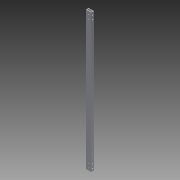
# Autodesk Inventor part: M - 26 inch rail
Saved by Autodesk Inventor 2013 (Build 170138000, 138)
## iProperties
Created: 2013-02-16
Part Number: M - 26 inch rail
Material: Aluminum 6061
Document SubType Name: Modeling
Designer: Moses
Mass: 356.175 g
Surface Area: 842.395 cm^2
Volume: 131.43 cm^3
Density: 2.71 g/cm^3
Author: Moses
Autodesk Inventor part; units mm, degrees
ref_plane "YZ Plane" through (0, 0, 0) normal (1, 0, 0) x (0, 1, 0)
ref_plane "XZ Plane" through (0, 0, 0) normal (0, 1, 0) x (-1, 0, 0)
sketch "Sketch1" plane through (0, 0, 0) normal (0, 1, 0) x (-1, 0, 0)
  line L0 (0, 0) -> (25.4, 0)
  line L1 (25.4, 0) -> (25.4, 12.7)
  line L2 (25.4, 12.7) -> (0, 12.7)
  line L3 (0, 12.7) -> (0, 0)
  line L4 (3.175, 9.525) -> (22.225, 9.525)
  line L5 (22.225, 9.525) -> (22.225, 3.175)
  line L6 (22.225, 3.175) -> (3.175, 3.175)
  line L7 (3.175, 3.175) -> (3.175, 9.525)
  dimension "d0" = 25.4
  dimension "d2" = 3.175
  dimension "d5" = 12.7
  constraints: 16 end point, 4 parallel, 2 perpendicular, 1 horizontal, 3 other
  measures "d0" distance of L1.end L2.end
  measures "d2" distance between parallel lines of L2 L4
  measures "d5" distance of L0.end L1.end
extrude "Extrusion1" add sketch "Sketch1" along normal blind 660.4
sketch "Sketch2" plane through (-25.4, 0, 12.7) normal (0, 0, 1) x (1, 0, 0)
  circle A0 centre (12.7, 41.275) radius 3.3782 projected
  circle A1 centre (12.7, 22.225) radius 3.3782 projected
  circle A2 centre (12.7, 619.125) radius 3.3782 projected
  circle A3 centre (12.7, 638.175) radius 3.3782 projected
  line L0 (25.4, 0) -> (0, 0) projected
  line L1 (25.4, 660.4) -> (25.4, 0) projected
  line L2 (0, 660.4) -> (25.4, 660.4) projected
  line L3 (0, 0) -> (0, 660.4) projected
extrude "Extrusion2" cut sketch "Sketch2" against normal blind 25.4 contours A0 | A1 | A2 | A3
ref_plane "Work Plane1" through (-25.4, 0, 6.35) normal (0, 0, 1) x (1, 0, 0)
sketch "Sketch3" plane through (0, 0, 0) normal (1, 0, 0) x (0, 0, -1)
  line L0 (-12.7, 0) -> (0, 0) projected
  line L1 (-12.7, 660.4) -> (0, 660.4) projected
  line L2 (-6.35, 0) -> (-6.35, 660.4) construction
  circle A0 centre (-6.35, 647.7) radius 3.175
  circle A1 centre (-6.35, 628.65) radius 3.175
  circle A2 centre (-6.35, 12.7) radius 3.175
  circle A3 centre (-6.35, 31.75) radius 3.175
  dimension "d8" = 6.35
  dimension "d10" = 12.7
  dimension "d11" = 19.05
  dimension "d12" = 12.7
  dimension "d13" = 19.05
  constraints: 4 centre point, 4 point on line, 3 equal radius, 2 end point, 2 midpoint
  measures "d8" diameter of A0
  measures "d10" distance of L2.start A2.centre
  measures "d11" distance of A2.centre A3.centre
  measures "d12" distance from line of L1 A0.centre
  measures "d13" distance of A0.centre A1.centre
extrude "Extrusion3" cut sketch "Sketch3" against normal blind 25.4
body "Solid1"
